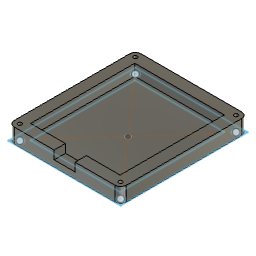
base (Autodesk Fusion 360 design; units mm, degrees)
Autodesk Fusion 360 part; units mm, degrees
sketch "Sketch1" plane through (0, 0, 0) normal (0, 0, 1) x (1, 0, 0)
  line L0 (-27.1259, 29.8327) -> (51.8741, 29.8327)
  line L1 (51.8741, 29.8327) -> (51.8741, -62.1673)
  line L2 (51.8741, -62.1673) -> (-27.1259, -62.1673)
  line L3 (-27.1259, -62.1673) -> (-27.1259, 29.8327)
  line L4 (62.3741, -72.1673) -> (-36.6259, -72.1673)
  line L5 (-36.6259, -72.1673) -> (-36.6259, 39.8327)
  line L6 (-36.6259, 39.8327) -> (62.3741, 39.8327)
  line L7 (62.3741, 39.8327) -> (62.3741, -72.1673)
  line L8 (62.3741, -72.1673) -> (-36.6259, 39.8327) construction
  line L9 (-36.6259, -72.1673) -> (62.3741, 39.8327) construction
  circle A0 centre (-31.6259, -67.1673) radius 1.7
  circle A1 centre (-31.6259, 34.8327) radius 1.7
  circle A2 centre (57.3741, 34.8327) radius 1.7
  circle A3 centre (57.3741, -67.1673) radius 1.7
  circle A4 centre (-31.6259, 34.8327) radius 3
  circle A5 centre (57.3741, 34.8327) radius 3
  circle A6 centre (57.3741, -67.1673) radius 3
  circle A7 centre (-31.6259, -67.1673) radius 3
  point P0 (12.8741, -16.1673)
  dimension "d1" = 79
  dimension "d3" = 99
  dimension "d4" = 112
  dimension "d13" = 3.4
  dimension "d14" = 5
  dimension "d15" = 5
  dimension "d16" = 9.5
  dimension "d17" = 6
  dimension "d18" = 6
  dimension "d19" = 6
  dimension "d20" = 6
  constraint horizontal L0
  constraint vertical L1
  constraint horizontal L2
  constraint vertical L3
  constraint horizontal L4
  constraint perpendicular L4 L5
  constraint parallel L4 L6
  constraint parallel L5 L7
  constraint coincident L8 P0
  constraint coincident L9 P0
  constraint concentric A1 A4
  constraint concentric A2 A5
  constraint concentric A3 A6
  constraint concentric A0 A7
  measures "d1" distance of L0.start L0.end
  measures "d3" distance of L5.end L6.end
  measures "d4" distance of L4.end L5.end
  measures "d13" diameter of A0
  measures "d14" distance of L4 A0.centre
  measures "d15" distance of L5 A0.centre
  measures "d16" distance of L3 L5
  measures "d17" diameter of A4
  measures "d18" diameter of A5
  measures "d19" diameter of A6
  measures "d20" diameter of A7
extrude "Extrude1" add sketch "Sketch1" along normal blind 9.9 from surface at 3.1 contours A4 | A5 | A6 | A7 makes body 1 at (-34.6222, 34.6832, 9.7) makes body 2 at (-34.3904, -68.3326, 9.7) makes body 3 at (54.3778, 34.6832, 9.7) makes body 4 at (54.8142, -68.7316, 9.7)
extrude "Extrude2" add sketch "Sketch1" along normal blind 13 contours L4 L5 L6 L7 bodies 1 2 3 4
extrude "Extrude3" add sketch "Sketch1" along normal blind 3 contours L0 L1 L2 L3 bodies 1
sketch "Sketch2" plane through (0, 0, 13) normal (0, 0, 1) x (-1, 0, 0)
  circle A0 centre (31.6259, -34.8327) radius 1.7
  circle A1 centre (-57.3741, 67.1673) radius 1.7
  line L0 (-51.8741, 62.1673) -> (27.1259, 62.1673)
  line L1 (27.1259, 62.1673) -> (27.1259, -29.8327)
  line L2 (27.1259, -29.8327) -> (-51.8741, -29.8327)
  line L3 (-51.8741, -29.8327) -> (-51.8741, 62.1673)
  line L4 (-62.3741, -39.8327) -> (36.6259, -39.8327)
  line L5 (36.6259, -39.8327) -> (36.6259, 72.1673)
  line L6 (36.6259, 72.1673) -> (-62.3741, 72.1673)
  line L7 (-62.3741, 72.1673) -> (-62.3741, -39.8327)
  circle A2 centre (31.6259, 67.1673) radius 1.7
  circle A3 centre (-57.3741, -34.8327) radius 1.7
  line L8 (-3.6241, 62.1673) -> (-22.1241, 62.1673)
  line L9 (-22.1241, 62.1673) -> (-22.1241, 72.1673)
  line L10 (-22.1241, 72.1673) -> (-3.6241, 72.1673)
  line L11 (-3.6241, 72.1673) -> (-3.6241, 62.1673)
  line L12 (-3.6241, 62.1673) -> (-22.1241, 72.1673) construction
  line L13 (-22.1241, 62.1673) -> (-3.6241, 72.1673) construction
  point P0 (-12.8741, 67.1673)
  dimension "d28" = 18.5
  constraint horizontal L8
  constraint perpendicular L8 L9
  constraint parallel L8 L10
  constraint parallel L9 L11
  constraint coincident L12 P0
  constraint coincident L13 P0
  measures "d28" distance of L9.end L10.end
extrude "Extrude4" cut sketch "Sketch2" against normal blind 7.5 contours L0 L6 L8 L9 L10 L11 bodies 1
fillet "Fillet1" radius 5 1 edges at (-36.6259, 39.8327, 6.5) on bodies 1
fillet "Fillet2" radius 5 3 edges at (62.3741, 39.8327, 6.5) (62.3741, -72.1673, 6.5) (-36.6259, -72.1673, 6.5) on bodies 1
